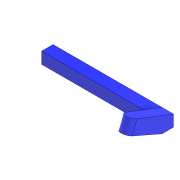
# Autodesk Inventor part: Radius_Bone1_Joint_LOWER
Saved by Autodesk Inventor 2020 (Build 240168000, 168)
## iProperties
Created: 2021-03-04
Part Number: Radius_Bone1_Joint_LOWER
Material: Generic
Document SubType Name: Modeling
Designer: deox
Density: 1 g/cm^3
Appearance: Blue - Wall Paint - Glossy
Author: deox
Autodesk Inventor part; units mm, degrees
ref_plane "YZ Plane" through (0, 0, 0) normal (1, 0, 0) x (0, 1, 0)
ref_plane "XZ Plane" through (0, 0, 0) normal (0, 1, 0) x (-1, 0, 0)
ref_plane "XY Plane" through (0, 0, 0) normal (0, 0, 1) x (1, 0, 0)
sketch "Sketch1" plane through (0, 0, 0) normal (1, 0, 0) x (0, 1, 0)
  line L0 (0, 0) -> (2.696, 0)
  line L1 (2.696, 0) -> (2.696, 6.6)
  circle A0 centre (2.696, 6.6) radius 0.5
  line L2 (-0.5, 0.5) -> (0.5, 0.5)
  line L3 (0.5, 0.5) -> (0.5, -0.5)
  line L4 (0.5, -0.5) -> (-0.5, -0.5)
  line L5 (-0.5, -0.5) -> (-0.5, 0.5)
  line L6 (-0.5, 0.5) -> (0.5, -0.5) construction
  line L7 (0.5, 0.5) -> (-0.5, -0.5) construction
  line L8 (0.5, -0.5) -> (3.1627, 6.4205)
  line L9 (-0.5, 0.5) -> (2.2374, 6.7993)
  dimension "d0" = 2.696
  dimension "d1" = 6.6
  dimension "d2" = 1
  dimension "d3" = 1
  dimension "d4" = 1
  constraints: 20 end point, 2 horizontal, 2 midpoint, 2 parallel, 2 perpendicular, 2 point on circle, 2 tangent, 1 centre point, 1 coincident
  measures "d0" distance of L0.start L0.end
  measures "d1" distance of L0.end L1.end
  measures "d2" diameter of A0
  measures "d3" distance of L3.end L4.end
  measures "d4" distance of L2.end L3.end
extrude "Extrusion1" add sketch "Sketch1" along normal blind 1 contours L3 L2 L9 A0 L1 L8 L0 | L3 L4 L5 L2 | L0 L8 L3 | L1 A0 L8 | A0
sketch "Sketch2" plane through (0, 0, 0) normal (-1, 0, 0) x (0, 0, 1)
  line L0 (-0.5, -0.5) -> (0.5, -0.5)
  line L1 (0.5, -0.5) -> (0.5, 0.5)
  line L2 (0.5, 0.5) -> (-0.5, 0.5)
  line L3 (-0.5, 0.5) -> (-0.5, -0.5)
  line L4 (-0.5, -0.5) -> (0.5, 0.5) construction
  line L5 (0.5, -0.5) -> (-0.5, 0.5) construction
  arc A0 (6.7993, 2.2374) -> (6.4205, 3.1627) centre (6.6, 2.696) ccw projected
  circle A1 centre (6.6, 2.696) radius 0.5
  point P0 (0, 0)
  point P1 (6.4205, 3.1627)
  point P2 (6.7993, 2.2374)
  dimension "d7" = 1
  dimension "d8" = 1
  constraints: 12 end point, 2 midpoint, 2 parallel, 1 centre point, 1 coincident, 1 horizontal, 1 perpendicular
  measures "d7" distance of L2.end L1.end
  measures "d8" distance of L1.end L0.end
extrude "Extrusion2" add sketch "Sketch2" along normal blind 9.53
sketch "Sketch3" plane through (0, 3.1627, 6.4205) normal (0, 0.9333, -0.3591) x (1, 0, 0)
  line L0 (0, 0) -> (1, 0) projected
  line L1 (1, 0) -> (1, 4)
  line L2 (1, 7.415) -> (1, 0) projected
  line L3 (1, 4) -> (0, 4)
  circle A0 centre (0.5, 4) radius 0.5
  line L4 (1, 4) -> (1.9656, 2.6006)
  line L5 (1.9656, 2.6006) -> (1.9656, -0.469)
  line L6 (1.9656, -0.469) -> (1.3988, -1.3966)
  line L7 (1.3988, -1.3966) -> (-6.1023, -1.6689)
  line L8 (-6.1023, -1.6689) -> (-10.3351, -1.4334)
  line L9 (-10.3351, -1.4334) -> (-10.659, 1.386)
  line L10 (-10.659, 1.386) -> (-5.3662, 3.1822)
  line L11 (-5.3662, 3.1822) -> (0, 4)
  point P0 (0, 7.1279)
  point P1 (1, 4)
  dimension "d11" = 4
  constraints: 20 end point, 1 midpoint, 1 perpendicular, 1 point on line, 1 vertical, 3 other
  measures "d11" distance of L0.end L1.end
extrude "Extrusion3" cut sketch "Sketch3" against normal blind 10 contours L4 L5 L6 L7 L8 L9 L10 L11 A0
body "Solid1"
